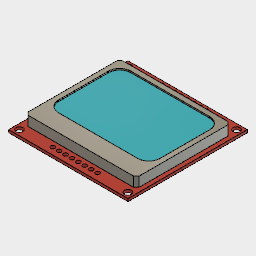
_Nokia 5110 LCD.51a67ab2-6302-4703-bf08-b63129d5c42c (Autodesk Fusion 360 design; units mm, degrees)
Autodesk Fusion 360 part; units mm, degrees
sketch "Sketch1" plane through (0, 0, 0) normal (0, 1, 0) x (1, 0, 0)
  line L0 (0, 0) -> (43, 0)
  line L1 (43, 0) -> (43, -43)
  line L2 (43, -43) -> (0, -43)
  line L3 (0, -43) -> (0, 0)
  dimension "d1" = 43
  dimension "d2" = 43
  measures "d1" distance of L0.start L0.end
  measures "d2" distance of L0.start L2.end L1
extrude "Extrude1" add sketch "Sketch1" along normal blind 1 makes body 1
copy_body "Body->Comp1" bodies 1 removing the originals makes body 2 in component "pcb"
sketch "Sketch1 (2)" plane through (0, 1, 0) normal (0, 1, 0) x (-1, 0, 0) in component "Component"
  line L0 (0, 43) -> (-43, 43)
  line L1 (-43, 43) -> (-43, 0)
  line L2 (-43, 0) -> (0, 0)
  line L3 (0, 0) -> (0, 43)
  line L4 (-1.5, 4.5) -> (-41.5, 4.5)
  line L5 (-41.5, 4.5) -> (-41.5, 38.5)
  line L6 (-41.5, 38.5) -> (-1.5, 38.5)
  line L7 (-1.5, 38.5) -> (-1.5, 4.5)
  dimension "d5" = 40
  dimension "d6" = 34
  dimension "d7" = 1.5
  dimension "d8" = 4.5
  measures "d5" distance of L4.start L4.end
  measures "d6" distance of L4.start L6.end
  measures "d7" distance of L3 L7
  measures "d8" distance of L2 L4
extrude "Extrude1'" add sketch "Sketch1 (2)" along normal blind 3.5 separate body contours L4 L5 L6 L7 makes body 3 in component "Component"
sketch "Sketch2" plane through (0, 4.5, 0) normal (0, 1, 0) x (-1, 0, 0) in component "Component"
  line L0 (-1.5, 38.5) -> (-41.5, 38.5)
  line L1 (-41.5, 38.5) -> (-41.5, 4.5)
  line L2 (-41.5, 4.5) -> (-1.5, 4.5)
  line L3 (-1.5, 4.5) -> (-1.5, 38.5)
  line L4 (-7.25, 6.25) -> (-35.75, 6.25)
  line L5 (-39.75, 10.25) -> (-39.75, 28.25)
  line L6 (-35.75, 32.25) -> (-7.25, 32.25)
  line L7 (-3.25, 28.25) -> (-3.25, 10.25)
  arc A0 (-7.25, 6.25) -> (-3.25, 10.25) centre (-7.25, 10.25) ccw
  arc A1 (-39.75, 10.25) -> (-35.75, 6.25) centre (-35.75, 10.25) ccw
  arc A2 (-35.75, 32.25) -> (-39.75, 28.25) centre (-35.75, 28.25) ccw
  arc A3 (-3.25, 28.25) -> (-7.25, 32.25) centre (-7.25, 28.25) ccw
  point P0 (-3.25, 6.25)
  point P1 (-39.75, 6.25)
  point P2 (-3.25, 32.25)
  dimension "d11" = 36.5
  dimension "d12" = 26
  dimension "d13" = 1.75
  dimension "d14" = 1.75
  dimension "d15" = 4
  measures "d11" distance of P0 P1
  measures "d12" distance of P0 P2
  measures "d13" distance of L3 L7
  measures "d14" distance of L2 L4
  measures "d15" radius of A0
extrude "Extrude2" cut sketch "Sketch2" against normal blind 0.5 contours L4 L5 L6 L7 A0 A1 A2 A3 bodies 3 in component "Component"
sketch "Sketch1 (3)" plane through (0, 1, 0) normal (0, 1, 0) x (-1, 0, 0) in component "pcb"
  line L0 (0, 43) -> (-43, 43)
  line L1 (-43, 43) -> (-43, 0)
  line L2 (-43, 0) -> (0, 0)
  line L3 (0, 0) -> (0, 43)
  circle A0 centre (-1.95, 1.95) radius 1.25
  circle A1 centre (-1.95, 41.05) radius 1.25
  circle A2 centre (-41.05, 41.05) radius 1.25
  circle A3 centre (-41.05, 1.95) radius 1.25
  point P0 (-21.5, 21.5)
  dimension "d18" = 2.5
  dimension "d19" = 1.95
  dimension "d20" = 1.95
  dimension "d22" = 360
  measures "d18" diameter of A0
  measures "d19" distance of L3 A0.centre
  measures "d20" distance of L2 A0.centre
extrude "Extrude1''" cut sketch "Sketch1 (3)" against normal up to surface (1 mm away) contours A0 | A1 | A2 | A3 bodies 2 in component "pcb"
sketch "Sketch2 (2)" plane through (0, 1, 0) normal (0, 1, 0) x (-1, 0, 0) in component "pcb"
  circle A0 centre (-41.05, 1.95) radius 1.25
  circle A1 centre (-41.05, 41.05) radius 1.25
  circle A2 centre (-1.95, 1.95) radius 1.25
  circle A3 centre (-1.95, 41.05) radius 1.25
  line L0 (0, 43) -> (-43, 43)
  line L1 (-43, 43) -> (-43, 0)
  line L2 (-43, 0) -> (0, 0)
  line L3 (0, 0) -> (0, 43)
  circle A4 centre (-13.45, 1.5) radius 0.75
  circle A5 centre (-15.75, 1.5) radius 0.75
  circle A6 centre (-18.05, 1.5) radius 0.75
  circle A7 centre (-20.35, 1.5) radius 0.75
  circle A8 centre (-22.65, 1.5) radius 0.75
  circle A9 centre (-24.95, 1.5) radius 0.75
  circle A10 centre (-27.25, 1.5) radius 0.75
  circle A11 centre (-29.55, 1.5) radius 0.75
  circle A12 centre (-13.45, 40.5) radius 0.75
  circle A13 centre (-15.75, 40.5) radius 0.75
  circle A14 centre (-18.05, 40.5) radius 0.75
  circle A15 centre (-20.35, 40.5) radius 0.75
  circle A16 centre (-22.65, 40.5) radius 0.75
  circle A17 centre (-24.95, 40.5) radius 0.75
  circle A18 centre (-27.25, 40.5) radius 0.75
  circle A19 centre (-29.55, 40.5) radius 0.75
  dimension "d25" = 1.5
  dimension "d26" = 1.5
  dimension "d29" = -2.3
  dimension "d30" = 39
  dimension "d31" = 13.45
  measures "d25" diameter of A4
  measures "d26" distance of L2 A4.centre
  measures "d31" distance of L1 A11.centre
extrude "Extrude2'" cut sketch "Sketch2 (2)" against normal through all contours A4 | A5 | A6 | A7 | A8 | A9 | A10 | A11 | A12 | A13 | A14 | A15 | A16 | A17 | A18 | A19 bodies 2 in component "pcb"
chamfer "Chamfer1" distance 1 angle 45 4 edges at (1.5, 2.75, 38.5) (1.5, 2.75, 4.5) (41.5, 2.75, 4.5) (41.5, 2.75, 38.5) on bodies 3 in component "Component"
sketch "Sketch3" plane through (0, 0, 0) normal (0, -1, 0) x (1, 0, 0) in component "Component"
  circle A0 centre (13.45, 40.5) radius 0.75
  circle A1 centre (22.65, 40.5) radius 0.75
  circle A2 centre (15.75, 1.5) radius 0.75
  circle A3 centre (27.25, 1.5) radius 0.75
  circle A4 centre (29.55, 1.5) radius 0.75
  circle A5 centre (18.05, 1.5) radius 0.75
  circle A6 centre (15.75, 40.5) radius 0.75
  circle A7 centre (20.35, 40.5) radius 0.75
  circle A8 centre (29.55, 40.5) radius 0.75
  circle A9 centre (24.95, 40.5) radius 0.75
  circle A10 centre (22.65, 1.5) radius 0.75
  circle A11 centre (24.95, 1.5) radius 0.75
  circle A12 centre (13.45, 1.5) radius 0.75
  circle A13 centre (20.35, 1.5) radius 0.75
  circle A14 centre (27.25, 40.5) radius 0.75
  circle A15 centre (18.05, 40.5) radius 0.75
  circle A16 centre (41.05, 1.95) radius 1.25
  circle A17 centre (41.05, 41.05) radius 1.25
  circle A18 centre (1.95, 1.95) radius 1.25
  circle A19 centre (1.95, 41.05) radius 1.25
  line L0 (43, 43) -> (0, 43)
  line L1 (0, 43) -> (0, 0)
  line L2 (0, 0) -> (43, 0)
  line L3 (43, 0) -> (43, 43)
  line L4 (39.8773, 6.3156) -> (40.8483, 6.5548)
  line L5 (40.8483, 6.5548) -> (40.0111, 9.9532)
  line L6 (40.0111, 9.9532) -> (39.0401, 9.714)
  line L7 (39.0401, 9.714) -> (39.8773, 6.3156)
  line L8 (3.8483, 6.5548) -> (3.0111, 9.9532)
  line L9 (2.0401, 9.714) -> (2.8773, 6.3156)
  line L10 (3.0111, 9.9532) -> (2.0401, 9.714)
  line L11 (2.8773, 6.3156) -> (3.8483, 6.5548)
  line L12 (40.8483, 33.5548) -> (40.0111, 36.9532)
  line L13 (39.0401, 36.714) -> (39.8773, 33.3156)
  line L14 (40.0111, 36.9532) -> (39.0401, 36.714)
  line L15 (39.8773, 33.3156) -> (40.8483, 33.5548)
  line L16 (3.8483, 33.5548) -> (3.0111, 36.9532)
  line L17 (2.0401, 36.714) -> (2.8773, 33.3156)
  line L18 (3.0111, 36.9532) -> (2.0401, 36.714)
  line L19 (2.8773, 33.3156) -> (3.8483, 33.5548)
  dimension "d34" = 3.5
  dimension "d35" = 1
  dimension "d38" = -37
  dimension "d39" = 27
  measures "d34" distance of L4.start L6.end
  measures "d35" distance of L4.start L4.end
extrude "Extrude3" add sketch "Sketch3" along normal blind 1.5 separate body contours L4 L5 L6 L7 | L8 L9 L10 L11 | L12 L13 L14 L15 | L16 L17 L18 L19 makes body 4 at (39.3192, -0.5, 35.5812) makes body 5 at (2.5982, -1, 7.4484) makes body 6 at (2.3192, -0.5, 35.5812) makes body 7 at (39.3192, -0.5, 8.5812) in component "Component"
component "pcb" placed x (1, 0, 0) y (0, 1, 0) z (0, 0, 1) at (0, 0, 0)
component "Component" placed x (1, 0, 0) y (0, 1, 0) z (0, 0, 1) at (0, 0, 0) in component "pcb"
equation "d7 = ( ( 43 - 40 ) / 2 ) * 1 mm"
equation "d8 = ( ( 43 - 34 ) / 2 ) * 1 mm"
equation "d13 = ( 40 mm - d11 ) / 2"
equation "d14 = d13"
equation "d19 = ( ( 2.5 / 2 ) + 0.7 ) * 1 mm"
